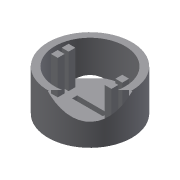
# Autodesk Inventor part: PI_holder
Saved by Autodesk Inventor 2014 (Build 180170000, 170)
## iProperties
Created: 2016-10-07
Part Number: PI_holder
Material: Generic
Document SubType Name: Modeling
Designer: Camilo
Density: 1 g/cm^3
Appearance: Default
Author: Camilo
Autodesk Inventor part; units mm, degrees
ref_plane "YZ Plane" through (0, 0, 0) normal (1, 0, 0) x (0, 1, 0)
ref_plane "XZ Plane" through (0, 0, 0) normal (0, 1, 0) x (-1, 0, 0)
ref_plane "XY Plane" through (0, 0, 0) normal (0, 0, 1) x (1, 0, 0)
sketch "Sketch1" plane through (0, 0, 0) normal (0, 0, 1) x (1, 0, 0)
  circle A0 centre (0, 0) radius 12.25 projected
  point P0 (0, 0)
extrude "Extrusion1" add sketch "Sketch1" along normal blind 2
sketch "Sketch2" plane through (0, 0, 2) normal (0, 0, 1) x (1, 0, 0)
  circle A0 centre (0, 0) radius 12.25 projected
  line L0 (-4.5, -0.75) -> (4.5, -0.75)
  line L1 (4.5, -0.75) -> (4.5, 0.75)
  line L2 (4.5, 0.75) -> (-4.5, 0.75)
  line L3 (-4.5, 0.75) -> (-4.5, -0.75)
  line L4 (-4.5, -0.75) -> (4.5, 0.75) construction
  line L5 (4.5, -0.75) -> (-4.5, 0.75) construction
  dimension "d13" = 9
  dimension "d14" = 1.5
  constraints: 12 end point, 2 horizontal, 2 midpoint, 2 vertical
  measures "d13" distance of L1.end L2.end
  measures "d14" distance of L2.end L0.start
extrude "Extrusion2" cut sketch "Sketch2" against normal through all contours L3 L2 L1 L0
sketch "Sketch3" plane through (0, 0, 2) normal (0, 0, 1) x (1, 0, 0)
  circle A0 centre (0, 0) radius 12.25 projected
  circle A1 centre (0, 0) radius 10.25
  dimension "d4" = 2
  constraints: 1 centre point, 1 coincident
  measures "d4" radial gap between concentric circles of A0 A1
extrude "Extrusion3" add sketch "Sketch3" along normal blind 10
sketch "Sketch4" plane through (0, 0, 2) normal (0, 0, 1) x (1, 0, 0)
  circle A0 centre (0, 0) radius 10.25 construction
  line L0 (-5.235, -0.75) -> (-8.355, -0.75) construction
  line L1 (-5.235, -1.51) -> (-8.355, -1.51) construction
  line L2 (-8.355, -0.75) -> (-8.355, -1.51) projected
  line L3 (-8.855, -0.55) -> (-6.855, -0.55)
  line L4 (-6.855, -0.55) -> (-6.855, 1.45)
  line L5 (-6.855, 1.45) -> (-8.855, 1.45)
  line L6 (-8.855, 1.45) -> (-8.855, -0.55)
  line L7 (-8.855, -0.55) -> (-6.855, 1.45) construction
  line L8 (-6.855, -0.55) -> (-8.855, 1.45) construction
  line L9 (-8.355, -1.13) -> (-6.0393, -1.13) construction
  line L10 (-8.855, -1.71) -> (-6.855, -1.71)
  line L11 (-6.855, -1.71) -> (-6.855, -3.71)
  line L12 (-6.855, -3.71) -> (-8.855, -3.71)
  line L13 (-8.855, -3.71) -> (-8.855, -1.71)
  line L14 (-8.855, -1.71) -> (-6.855, -3.71) construction
  line L15 (-6.855, -1.71) -> (-8.855, -3.71) construction
  line L16 (0, 0) -> (0, -2.4826) construction
  line L17 (8.855, -0.55) -> (6.855, -0.55)
  line L18 (6.855, -0.55) -> (6.855, 1.45)
  line L19 (6.855, 1.45) -> (8.855, 1.45)
  line L20 (8.855, 1.45) -> (8.855, -0.55)
  line L21 (8.855, -0.55) -> (6.855, 1.45) construction
  line L22 (6.855, -0.55) -> (8.855, 1.45) construction
  line L23 (6.855, -1.71) -> (6.855, -3.71)
  line L24 (8.855, -1.71) -> (6.855, -1.71)
  line L25 (6.855, -3.71) -> (8.855, -3.71)
  line L26 (8.855, -1.71) -> (6.855, -3.71) construction
  line L27 (6.855, -1.71) -> (8.855, -3.71) construction
  line L28 (8.855, -3.71) -> (8.855, -1.71)
  point P0 (-7.855, 0.45)
  point P1 (-7.855, -2.71)
  point P2 (7.855, 0.45)
  point P3 (7.855, -2.71)
  dimension "d7" = 0.2
  dimension "d8" = 0.5
  dimension "d9" = 2
  dimension "d10" = 2
  constraints: 52 end point, 15 symmetric about line, 9 midpoint, 1 horizontal, 1 vertical
  measures "d7" distance between parallel lines of L0 L3
  measures "d8" distance between parallel lines of L2 L6
  measures "d9" distance of L4.end L5.end
  measures "d10" distance of L3.end L4.end
extrude "Extrusion4" add sketch "Sketch4" along normal up to surface (10 mm away)
body "Solid1"
